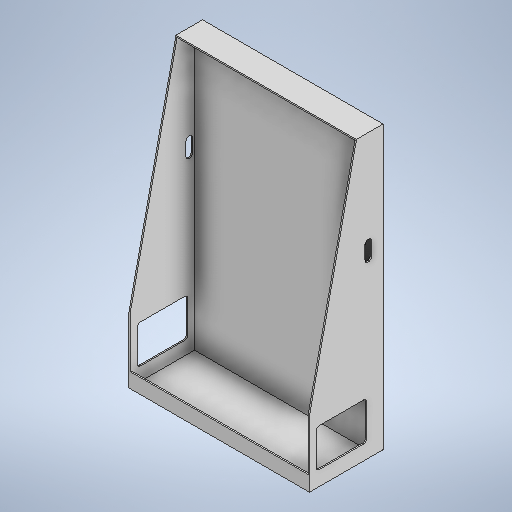
# Autodesk Inventor part: Стенд
Saved by Autodesk Inventor 2025 (Build 290162010, 162A)
## iProperties
Created: 2025-11-19
Part Number: Стенд
Material: Generic
Document SubType Name: Modeling
Designer: pokla
Density: 1 g/cm^3
Appearance: Default
Author: pokla
Autodesk Inventor part; units mm, degrees
ref_plane "YZ Plane" through (0, 0, 0) normal (1, 0, 0) x (0, 1, 0)
ref_plane "XZ Plane" through (0, 0, 0) normal (0, 1, 0) x (-1, 0, 0)
ref_plane "XY Plane" through (0, 0, 0) normal (0, 0, 1) x (1, 0, 0)
sketch "Sketch1" plane through (0, 0, 0) normal (1, 0, 0) x (0, 1, 0)
  line L0 (0, 0) -> (-550, 0)
  line L1 (0, 0) -> (0, 2110)
  line L2 (-550, 0) -> (-550, 495)
  line L3 (-550, 495) -> (-200, 2100)
  line L4 (0, 2110) -> (-200, 2110)
  line L5 (-200, 2110) -> (-200, 2100)
  line L6 (-475, 395) -> (-145, 395)
  line L7 (-120, 370) -> (-120, 135)
  line L8 (-145, 110) -> (-475, 110)
  line L9 (-500, 135) -> (-500, 370)
  arc A0 (-475, 395) -> (-500, 370) centre (-475, 370) ccw
  arc A1 (-500, 135) -> (-475, 110) centre (-475, 135) ccw
  arc A2 (-145, 110) -> (-120, 135) centre (-145, 135) ccw
  arc A3 (-120, 370) -> (-145, 395) centre (-145, 370) ccw
  line L10 (-110, 1420) -> (-110, 1420)
  line L11 (-85, 1395) -> (-85, 1295)
  line L12 (-110, 1270) -> (-110, 1270)
  line L13 (-135, 1295) -> (-135, 1395)
  arc A4 (-110, 1420) -> (-135, 1395) centre (-110, 1395) ccw
  arc A5 (-85, 1395) -> (-110, 1420) centre (-110, 1395) ccw
  arc A6 (-110, 1270) -> (-85, 1295) centre (-110, 1295) ccw
  arc A7 (-135, 1295) -> (-110, 1270) centre (-110, 1295) ccw
  point P0 (-120, 110)
  point P1 (-500, 110)
  point P2 (-85, 1270)
  point P3 (-85, 1420)
  point P4 (-135, 1270)
  dimension "d0" = 550
  dimension "d1" = 2110
  dimension "d2" = 495
  dimension "d3" = 200
  dimension "d4" = 10
  dimension "d5" = 380
  dimension "d6" = 285
  dimension "d10" = 110
  dimension "d11" = 120
  dimension "d12" = 25
  dimension "d13" = 50
  dimension "d14" = 150
  dimension "d15" = 1270
  dimension "d16" = 85
  dimension "d17" = 25
  constraints: 28 end point, 16 point on circle, 16 tangent, 10 point on line, 8 centre point, 6 equal radius, 4 horizontal, 4 parallel, 3 vertical, 2 perpendicular
  measures "d0" distance of L0.start L0.end
  measures "d1" distance of L0.start L1.end
  measures "d2" distance of L0.end L2.end
  measures "d3" distance of L1.end L4.end
  measures "d4" distance of L4.end L3.end
  measures "d5" distance of point (-120, 110) point (-500, 110)
  measures "d6" distance between parallel lines of L6 L8
  measures "d10" distance between parallel lines of L0 L8
  measures "d11" distance between parallel lines of L7 L1
  measures "d12" radius of A0
  measures "d13" distance of point (-85, 1270) point (-135, 1270)
  measures "d14" distance of point (-85, 1420) point (-85, 1270)
  measures "d15" distance between parallel lines of L0 L12
  measures "d16" distance between parallel lines of L1 L11
  measures "d17" radius of A4
extrude "Extrusion1" add sketch "Sketch1" along normal mid plane 1350
sketch "Sketch2" plane through (-675, 0, 2110) normal (0, 1, 0) x (1, 0, 0)
  line L0 (1340, 10) -> (10, 10)
  line L1 (10, 10) -> (10, 2110)
  line L2 (10, 2110) -> (1340, 2110)
  line L3 (1340, 2110) -> (1340, 10)
  line L4 (0, 0) -> (1350, 0) projected
  line L5 (1350, 2110) -> (1350, 0) projected
  line L6 (0, 0) -> (0, 2110) projected
  line L7 (0, 2110) -> (1350, 2110) projected
  point P0 (675, 2110)
  dimension "d20" = 10
  dimension "d21" = 10
  dimension "d22" = 10
  dimension "d23" = 0
  constraints: 8 end point, 2 parallel, 1 horizontal, 1 perpendicular
  measures "d20" distance between parallel lines of L4 L0
  measures "d21" distance between parallel lines of L5 L3
  measures "d22" distance between parallel lines of L6 L1
  measures "d23" distance between parallel lines of L7 L2
extrude "Extrusion2" cut sketch "Sketch2" against normal blind 60 contours L0 L1 L2 L3
sketch "Sketch3" plane through (-675, -550, 0) normal (0, -1, 0) x (1, 0, 0)
  line L0 (10, 2100) -> (1340, 2100)
  line L1 (1340, 2100) -> (1340, 110)
  line L2 (1340, 110) -> (10, 110)
  line L3 (10, 110) -> (10, 2100)
  line L4 (1350, 2100) -> (1350, 495) projected
  line L5 (0, 495) -> (0, 2100) projected
  line L6 (1350, 2110) -> (0, 2110) projected
  line L7 (0, 0) -> (1350, 0) projected
  point P0 (675, 0)
  dimension "d26" = 10
  dimension "d27" = 10
  dimension "d28" = 10
  dimension "d29" = 110
  constraints: 8 end point, 2 parallel, 1 horizontal, 1 perpendicular
  measures "d26" distance between parallel lines of L4 L1
  measures "d27" distance between parallel lines of L5 L3
  measures "d28" distance between parallel lines of L6 L0
  measures "d29" distance between parallel lines of L7 L2
extrude "Extrusion3" cut sketch "Sketch3" against normal blind 480
sketch "Sketch4" plane through (675, -475, 110) normal (0, 0, 1) x (1, 0, 0)
  line L0 (-1340, -65) -> (-10, -65)
  line L1 (-10, -65) -> (-10, 405)
  line L2 (-10, 405) -> (-1340, 405)
  line L3 (-1340, 405) -> (-1340, -65)
  line L4 (-1350, -75) -> (-1350, 275) projected
  line L5 (-10, -75) -> (-1340, -75) projected
  line L6 (0, 275) -> (0, -75) projected
  line L7 (-1340, 415) -> (-10, 415) projected
  point P0 (-675, 475)
  dimension "d32" = 10
  dimension "d33" = 10
  dimension "d34" = 10
  dimension "d35" = 10
  constraints: 8 end point, 2 parallel, 1 horizontal, 1 perpendicular
  measures "d32" distance between parallel lines of L4 L3
  measures "d33" distance between parallel lines of L5 L0
  measures "d34" distance between parallel lines of L6 L1
  measures "d35" distance between parallel lines of L7 L2
extrude "Extrusion4" cut sketch "Sketch4" against normal blind 100
body "Solid1"
